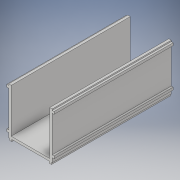
# Autodesk Inventor part: CompactSlidePart2
Saved by Autodesk Inventor 2017 (Build 210142000, 142)
## iProperties
Created: 2017-11-11
Part Number: CompactSlidePart2
Material: Generic
Document SubType Name: Modeling
Designer: User
Density: 1 g/cm^3
Appearance: Default
Author: User
Autodesk Inventor part; units mm, degrees
ref_plane "YZ Plane" through (0, 0, 0) normal (1, 0, 0) x (0, 1, 0)
ref_plane "XZ Plane" through (0, 0, 0) normal (0, 1, 0) x (-1, 0, 0)
ref_plane "XY Plane" through (0, 0, 0) normal (0, 0, 1) x (1, 0, 0)
sketch "Sketch1" plane through (0, 0, 0) normal (0, 0, 1) x (1, 0, 0)
  line L0 (111.125, 0) -> (104.775, 0)
  line L1 (104.775, 0) -> (104.775, -112.7125)
  line L2 (104.775, -112.7125) -> (6.35, -112.7125)
  line L3 (6.35, -112.7125) -> (6.35, 0)
  line L4 (6.35, 0) -> (0, 0)
  line L5 (0, 0) -> (0, -3.175)
  line L6 (0, -3.175) -> (-4.7752, -3.175)
  line L7 (-4.7752, -3.175) -> (-4.7752, -9.525)
  line L8 (-4.7752, -9.525) -> (0, -9.525)
  line L9 (0, -119.0625) -> (0, -107.9373)
  line L10 (0, -107.9373) -> (-4.7752, -107.9373)
  line L11 (-4.7752, -107.9373) -> (-4.7752, -101.5873)
  line L12 (-4.7752, -101.5873) -> (0, -101.5873)
  line L13 (0, -119.0625) -> (1.5875, -119.0625)
  line L14 (1.5875, -119.0625) -> (1.5875, -123.8377)
  line L15 (1.5875, -123.8377) -> (7.9375, -123.8377)
  line L16 (7.9375, -123.8377) -> (7.9375, -119.0625)
  line L17 (0, 0) -> (0, -3.175)
  line L18 (0, -9.525) -> (0, -101.5873)
  line L19 (0, -107.9373) -> (0, -119.0625)
  line L20 (0, -119.0625) -> (1.5875, -119.0625)
  line L21 (111.125, -3.175) -> (115.9002, -3.175)
  line L22 (115.9002, -3.175) -> (115.9002, -9.525)
  line L23 (115.9002, -9.525) -> (111.125, -9.525)
  line L24 (111.125, -3.175) -> (111.125, 0)
  line L25 (111.125, -107.9373) -> (115.9002, -107.9373)
  line L26 (115.9002, -107.9373) -> (115.9002, -101.5873)
  line L27 (115.9002, -101.5873) -> (111.125, -101.5873)
  line L28 (111.125, -119.0625) -> (111.125, -107.9373)
  line L29 (111.125, -101.5873) -> (111.125, -9.525)
  line L30 (111.125, -119.0625) -> (109.5375, -119.0625)
  line L31 (109.5375, -119.0625) -> (109.5375, -123.8377)
  line L32 (109.5375, -123.8377) -> (103.1875, -123.8377)
  line L33 (103.1875, -123.8377) -> (103.1875, -119.0625)
  line L34 (7.9375, -119.0625) -> (103.1875, -119.0625)
  line L35 (109.5375, -119.0625) -> (111.125, -119.0625)
  dimension "d0" = 119.0625
  dimension "d1" = 111.125
  dimension "d2" = 6.35
  dimension "d3" = 112.7125
  dimension "d4" = 98.425
  dimension "d7" = 119.0625
  dimension "d10" = 3.175
  dimension "d11" = 4.7752
  dimension "d12" = 6.35
  dimension "d13" = 11.1252
  dimension "d14" = 4.7752
  dimension "d15" = 6.35
  dimension "d16" = 1.5875
  dimension "d17" = 4.7752
  dimension "d18" = 6.35
  dimension "d19" = 4.7752
  dimension "d20" = 4.7752
  dimension "d21" = 1.5875
  dimension "d22" = 6.35
  dimension "d23" = 6.35
  constraints: 72 end point, 45 perpendicular, 6 parallel, 4 horizontal, 3 vertical, 1 point on line
  measures "d0" distance of L4.end L9.start
  measures "d1" distance of L9.start L28.start
  measures "d2" distance of L0.start L0.end
  measures "d3" distance of L0.end L1.end
  measures "d4" distance of L1.end L2.end
  measures "d7" distance of L28.start L0.start
  measures "d10" distance of L4.end L5.end
  measures "d11" distance of L5.end L6.end
  measures "d12" distance of L6.end L7.end
  measures "d13" distance of L9.start L9.end
  measures "d14" distance of L9.end L10.end
  measures "d15" distance of L10.end L11.end
  measures "d16" distance of L9.start L13.end
  measures "d17" distance of L13.end L14.end
  measures "d18" distance of L14.end L15.end
  measures "d19" distance of L21.start L21.end
  measures "d20" distance of L25.start L25.end
  measures "d21" distance of L28.start L30.end
  measures "d22" distance of L31.end L32.end
  measures "d23" distance between parallel lines of L3 L5
extrude "Extrusion1" add sketch "Sketch1" along normal blind 304.8
body "Solid1"
